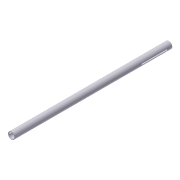
# Autodesk Inventor part: FE-00028
Saved by Autodesk Inventor 2012 (Build 160160000, 160)
## iProperties
Created: 2008-05-24
Part Number: FE-00028
Document SubType Name: Modeling
Designer: firstuser
Density: 1 g/cm^3
Description: Arm, Field Gate
Mass: 412.018 g
Surface Area: 2333.16 cm^2
Volume: 412.018 cm^3
Material: Default
Author: firstuser
Autodesk Inventor part; units mm, degrees
ref_plane "XZ Plane" through (0, 0, 0) normal (0, 1, 0) x (-1, 0, 0)
ref_plane "XY Plane" through (0, 0, 0) normal (0, 0, 1) x (1, 0, 0)
sketch "Sketch1" plane through (0, 0, 0) normal (0, 0, 1) x (1, 0, 0)
  circle A0 centre (0, 0) radius 21.0312
  circle A1 centre (0, 0) radius 17.4625
  dimension "d0" = 42.0624
  dimension "d1" = 34.925
  constraints: 2 centre point, 1 coincident
  measures "d0" diameter of A0
  measures "d1" diameter of A1
extrude "Extrusion1" add sketch "Sketch1" along normal mid plane 965.2
ref_plane "Work Plane1" through (0, 0, 0) normal (1, 0, 0) x (0, 0, 1)
sketch "Sketch2" plane through (0, 0, 0) normal (1, 0, 0) x (0, 0, 1)
  line L0 (-482.6, -21.0312) -> (482.6, -21.0312) projected
  line L1 (-482.6, 21.0312) -> (482.6, 21.0312) projected
  line L2 (482.6, 17.4625) -> (482.6, -17.4625) projected
  line L3 (482.6, 21.0312) -> (482.6, -21.0312) projected
  line L4 (-482.6, -17.4625) -> (-482.6, 17.4625) projected
  line L5 (-482.6, -21.0312) -> (-482.6, 21.0312) projected
  line L6 (-675.64, 0) -> (675.64, 0) projected
  arc A0 (474.6625, -3.175) -> (474.6625, 3.175) centre (474.6625, 0) ccw
  arc A1 (436.5625, -3.175) -> (436.5625, 3.175) centre (436.5625, 0) ccw
  arc A2 (461.9625, 3.175) -> (461.9625, -3.175) centre (461.9625, 0) ccw
  arc A3 (423.8625, 3.175) -> (423.8625, -3.175) centre (423.8625, 0) ccw
  line L7 (423.8625, 3.175) -> (436.5625, 3.175)
  line L8 (423.8625, -3.175) -> (436.5625, -3.175)
  line L9 (461.9625, -3.175) -> (474.6625, -3.175)
  line L10 (461.9625, 3.175) -> (474.6625, 3.175)
  dimension "d5" = 7.9375
  dimension "d6" = 38.1
  dimension "d7" = 6.35
  dimension "d18" = 12.7
  dimension "d19" = 12.7
  constraints: 8 end point, 8 point on circle, 6 tangent, 4 centre point, 4 point on line, 2 parallel, 1 equal radius
  measures "d5" distance from line of A0.centre L2
  measures "d6" distance of A1.centre A0.centre
  measures "d7" diameter of A0
  measures "d18" distance of A2.centre A0.centre
  measures "d19" distance of A3.centre A1.centre
extrude "Extrusion2" cut sketch "Sketch2" against normal blind 965.2 contours A3 L7 A1 L6 | L6 A1 L8 A3 | A0 L9 A2 L6 | L6 A2 L10 A0
sketch "Sketch3" plane through (0, 0, 0) normal (1, 0, 0) x (0, 0, 1)
  line L0 (-298.45, -3.175) -> (-450.85, -3.175)
  line L1 (-454.025, 0) -> (-454.025, 6.35)
  line L2 (-450.85, 9.525) -> (-450.85, 9.525)
  line L3 (-447.675, 6.35) -> (-447.675, 3.175)
  line L4 (-447.675, 3.175) -> (-298.45, 3.175)
  arc A0 (-298.45, -3.175) -> (-298.45, 3.175) centre (-298.45, 0) ccw
  arc A1 (-450.85, 9.525) -> (-454.025, 6.35) centre (-450.85, 6.35) ccw
  arc A2 (-447.675, 6.35) -> (-450.85, 9.525) centre (-450.85, 6.35) ccw
  arc A3 (-454.025, 0) -> (-450.85, -3.175) centre (-450.85, 0) ccw
  line L5 (-482.6, -21.0312) -> (-482.6, 21.0312) projected
  line L6 (-675.64, 0) -> (675.64, 0) projected
  dimension "d10" = 6.35
  dimension "d11" = 6.35
  dimension "d12" = 3.175
  dimension "d13" = 6.35
  dimension "d14" = 152.4
  dimension "d15" = 31.75
  constraints: 10 end point, 8 point on circle, 8 tangent, 4 centre point, 3 parallel, 1 concentric, 1 equal radius, 1 horizontal, 1 perpendicular, 1 point on line
  measures "d10" distance between parallel lines of L0 L4
  measures "d11" distance between parallel lines of L3 L1
  measures "d12" radius of A1
  measures "d13" distance of A1.centre A3.centre
  measures "d14" distance of A0.centre A3.centre
  measures "d15" distance from line of A1.centre L5
extrude "Extrusion3" cut sketch "Sketch3" along normal blind 965.2
body "Solid1"
